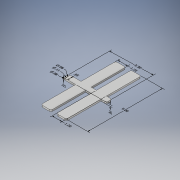
# Autodesk Inventor part: Grab Holder v1
Saved by Autodesk Inventor 2018 (Build 220112000, 112)
## iProperties
Created: 2019-12-06
Part Number: Grab Holder v1
Material: Generic
Document SubType Name: Modeling
Designer: AOFUser
Density: 1 g/cm^3
Appearance: Default
Author: AOFUser
Autodesk Inventor part; units mm, degrees
ref_plane "YZ Plane" through (0, 0, 0) normal (1, 0, 0) x (0, 1, 0)
ref_plane "XZ Plane" through (0, 0, 0) normal (0, 1, 0) x (-1, 0, 0)
ref_plane "XY Plane" through (0, 0, 0) normal (0, 0, 1) x (1, 0, 0)
sketch "Sketch1" plane through (0, 0, 0) normal (0, 1, 0) x (-1, 0, 0)
  line L0 (0, 0) -> (-134.62, 0)
  line L1 (-134.62, 0) -> (-134.62, -16.51)
  line L2 (-134.62, -16.51) -> (0, -16.51)
  line L3 (0, -16.51) -> (0, 0)
  line L4 (-134.62, -8.255) -> (-118.11, -8.255)
  line L5 (-118.11, -8.255) -> (-87.63, -8.255)
  line L6 (-87.63, -8.255) -> (-71.12, -8.255)
  line L7 (-71.12, -8.255) -> (-40.64, -8.255)
  line L8 (-40.64, -8.255) -> (-40.64, -122.555)
  line L9 (-40.64, -122.555) -> (-71.12, -122.555)
  line L10 (-71.12, -122.555) -> (-71.12, -8.255)
  line L11 (-87.63, -8.255) -> (-87.63, -122.555)
  line L12 (-87.63, -122.555) -> (-118.11, -122.555)
  line L13 (-118.11, -122.555) -> (-118.11, -8.255)
  line L14 (-118.11, -8.255) -> (-118.11, 106.045)
  line L15 (-118.11, 106.045) -> (-87.63, 106.045)
  line L16 (-87.63, 106.045) -> (-87.63, -8.255)
  line L17 (-71.12, -8.255) -> (-71.12, 106.045)
  line L18 (-71.12, 106.045) -> (-40.64, 106.045)
  line L19 (-40.64, 106.045) -> (-40.64, -8.255)
  dimension "d0" = 134.62
  dimension "d1" = 16.51
  dimension "d2" = 16.51
  dimension "d3" = 30.48
  dimension "d4" = 16.51
  dimension "d5" = 30.48
  dimension "d7" = 114.3
  dimension "d8" = 30.48
  dimension "d9" = 114.3
  dimension "d10" = 30.48
  dimension "d11" = 114.3
  dimension "d12" = 30.48
  dimension "d13" = 114.3
  dimension "d14" = 30.48
  constraints: 40 end point, 5 point on line, 3 horizontal, 3 perpendicular, 3 vertical, 2 parallel, 1 midpoint
  measures "d0" distance of L2.end L1.end
  measures "d1" distance of L1.end L0.end
  measures "d2" distance of L4.start L4.end
  measures "d3" distance of L4.end L5.end
  measures "d4" distance of L5.end L6.end
  measures "d5" distance of L6.end L7.end
  measures "d7" distance of L7.end L8.end
  measures "d8" distance of L8.end L9.end
  measures "d9" distance of L5.end L11.end
  measures "d10" distance of L11.end L12.end
  measures "d11" distance of L4.end L14.end
  measures "d12" distance of L14.end L15.end
  measures "d13" distance of L6.end L17.end
  measures "d14" distance of L17.end L18.end
extrude "Extrusion1" add sketch "Sketch1" along normal blind 5.08
fillet "Fillet1" radius 5.08 7 edges at (40.64, 2.54, -122.555) (71.12, 2.54, -122.555) (87.63, 2.54, -122.555) (118.11, 2.54, -122.555) (40.64, 2.54, 106.045) (87.63, 2.54, 106.045) (134.62, 2.54, -16.51)
fillet "Fillet2" radius 5.08 3 edges at (71.12, 2.54, 106.045) (118.11, 2.54, 106.045) (134.62, 2.54, 0)
sketch "Sketch2" plane through (0, 5.08, 0) normal (0, 1, 0) x (1, 0, 0)
  line L0 (40.64, 16.51) -> (0, 16.51) projected
  line L1 (0, 0) -> (8.128, 0)
  line L2 (8.128, 0) -> (8.128, 16.51)
  line L3 (8.128, 16.51) -> (0, 16.51)
  line L4 (0, 16.51) -> (0, 0)
  dimension "d19" = 8.128
  constraints: 8 end point, 2 parallel, 1 horizontal, 1 perpendicular, 1 point on line
  measures "d19" distance of L3.end L2.end
extrude "Extrusion2" cut sketch "Sketch2" against normal blind 3.81
sketch "Sketch3" plane through (0, 1.27, 0) normal (0, 1, 0) x (1, 0, 0)
  line L0 (0, 16.51) -> (0, 0) projected
  line L1 (0, 8.255) -> (3.81, 8.255)
  circle A0 centre (3.81, 8.255) radius 1.397
  line L2 (3.81, 0) -> (3.81, 3.81)
  line L3 (3.81, 16.51) -> (3.81, 12.7)
  circle A1 centre (3.81, 12.7) radius 1.016
  circle A2 centre (3.81, 3.81) radius 1.016
  dimension "d22" = 3.81
  dimension "d23" = 2.794
  dimension "d24" = 3.81
  dimension "d25" = 3.81
  dimension "d26" = 2.032
  dimension "d27" = 2.032
  constraints: 6 end point, 3 centre point, 3 coincident, 2 vertical, 1 horizontal, 1 midpoint
  measures "d22" distance of L1.start L1.end
  measures "d23" diameter of A0
  measures "d24" distance of L2.start L2.end
  measures "d25" distance of L3.start L3.end
  measures "d26" diameter of A1
  measures "d27" diameter of A2
extrude "Extrusion3" cut sketch "Sketch3" against normal blind 1.27
body "Solid1"
